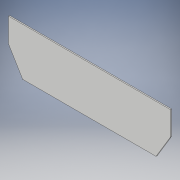
# Autodesk Inventor part: Inner Plate
Saved by Autodesk Inventor 2017 (Build 210142000, 142)
## iProperties
Created: 2017-10-13
Part Number: Inner Plate
Material: Generic
Document SubType Name: Modeling
Designer: Kenneth
Density: 1 g/cm^3
Appearance: Default
Author: Kenneth
Autodesk Inventor part; units mm, degrees
ref_plane "YZ Plane" through (0, 0, 0) normal (1, 0, 0) x (0, 1, 0)
ref_plane "XZ Plane" through (0, 0, 0) normal (0, 1, 0) x (-1, 0, 0)
ref_plane "XY Plane" through (0, 0, 0) normal (0, 0, 1) x (1, 0, 0)
sketch "Sketch1" plane through (0, 0, 0) normal (0, 0, 1) x (1, 0, 0)
  line L0 (-206.5357, 101.3775) -> (225.2643, 101.3775)
  line L1 (225.2643, 101.3775) -> (225.2643, 37.8775)
  line L2 (225.2643, 37.8775) -> (187.1643, -25.6225)
  line L3 (187.1643, -25.6225) -> (-168.4357, -25.6225)
  line L4 (-168.4357, -25.6225) -> (-206.5357, 37.8775)
  line L5 (-206.5357, 37.8775) -> (-206.5357, 101.3775)
  point P0 (0, 0)
  dimension "d0" = 431.8
  dimension "d1" = 355.6
  dimension "d2" = 63.5
  dimension "d3" = 90
  dimension "d5" = 63.5
  dimension "d7" = 63.5
  constraints: 12 end point, 1 horizontal, 1 parallel, 1 perpendicular
  measures "d0" distance of L0.start L0.end
  measures "d1" distance of L2.end L3.end
  measures "d2" distance of L4.end L0.start
  measures "d3" angle of L0 L5
  measures "d5" distance of L0.end L1.end
  measures "d7" vertical distance of L3.end L4.end
extrude "Extrusion1" add sketch "Sketch1" along normal blind 3.175
body "Solid1"
